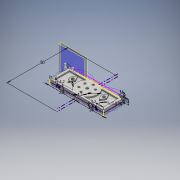
# Autodesk Inventor part: m_mount_l
Saved by Autodesk Inventor 2016 (Build 200138000, 138)
## iProperties
Created: 2016-12-01
Part Number: m_mount_l
Material: 一般
Document SubType Name: Modeling
Designer: KOTA-NPC2
Density: 1 g/cm^3
Appearance: 既定
Author: KOTA-NPC2
Autodesk Inventor part; units mm, degrees
ref_plane "YZ Plane" through (0, 0, 0) normal (1, 0, 0) x (0, 1, 0)
ref_plane "XZ Plane" through (0, 0, 0) normal (0, 1, 0) x (-1, 0, 0)
ref_plane "XY Plane" through (0, 0, 0) normal (0, 0, 1) x (1, 0, 0)
sketch "構築線" plane through (0, 0, 0) normal (0, 0, 1) x (1, 0, 0)
  circle A0 centre (0, 0) radius 8.5
  circle A1 centre (0, 0) radius 2.8 construction
  circle A2 centre (0, 0) radius 5 construction
  line L0 (0, -8.6) -> (-25, -8.6) construction
  line L1 (0, -11.6) -> (-25, -11.6) construction
  circle A3 centre (-12.8148, 0.95) radius 10.05 construction
  circle A4 centre (-12.8148, 0.95) radius 12.55 construction
  circle A5 centre (0, 5) radius 0.8
  circle A6 centre (-4.3301, 2.5) radius 0.8
  circle A7 centre (-4.3301, -2.5) radius 0.8
  circle A8 centre (0, -5) radius 0.8
  circle A9 centre (4.3301, -2.5) radius 0.8
  circle A10 centre (4.3301, 2.5) radius 0.8
  line L2 (25, -8.6) -> (0, -8.6) construction
  circle A11 centre (12.8148, 0.95) radius 10.05 construction
  circle A12 centre (12.8148, 0.95) radius 12.55 construction
  line L3 (0, -11.6) -> (25, -11.6) construction
  line L4 (-22, -8.6) -> (0, -8.6)
  line L5 (0, 25) -> (0, -25)
  line L6 (0, -8.6) -> (22, -8.6)
  circle A13 centre (0, 0) radius 3
  circle A14 centre (0, 0) radius 1
  circle A15 centre (12.8148, 0.95) radius 1.05
  circle A16 centre (-12.8148, 0.95) radius 1.05
  circle A17 centre (12.8148, 0.95) radius 2.75
  circle A18 centre (-12.8148, 0.95) radius 2.75
  line L7 (-4.8008, 7.0144) -> (-17, 7.0144)
  line L8 (4.8008, 7.0144) -> (17, 7.0144)
  line L9 (-4.8008, 7.0144) -> (4.8008, 7.0144)
  line L10 (-17, 7.0144) -> (-22, 7.0144)
  line L11 (-22, 7.0144) -> (-22, -8.6)
  line L12 (22, -8.6) -> (22, 7.0144)
  line L13 (22, 7.0144) -> (17, 7.0144)
  dimension "d22" = 20.1
  dimension "d41" = 20.1
  dimension "d0" = 17
  dimension "d1" = 5.6
  dimension "d2" = 10
  dimension "d12" = 25
  dimension "d13" = 8.6
  dimension "d14" = 0
  dimension "d17" = 0
  dimension "d18" = 25
  dimension "d19" = 3
  dimension "d23" = 25.1
  dimension "d29" = 1.6
  dimension "d30" = 0
  dimension "d31" = 5
  dimension "d34" = 360
  dimension "d38" = 25
  dimension "d42" = 25.1
  dimension "d43" = 25
  dimension "d46" = 22
  dimension "d49" = 50
  dimension "d50" = 25
  dimension "d51" = 25
  dimension "d52" = 22
  dimension "d58" = 6
  dimension "d59" = 2
  dimension "d99" = 2.1
  dimension "d100" = 2.1
  dimension "d105" = 5.5
  dimension "d106" = 5.5
  constraints: 28 end point, 17 centre point, 8 coincident, 8 horizontal, 2 perpendicular, 2 point on circle, 2 tangent, 2 vertical, 1 collinear, 1 concentric, 1 point on line, 23 other
  measures "d0" diameter of A0
  measures "d1" diameter of A1
  measures "d2" diameter of A2
  measures "d12" distance of L0.start L0.end
  measures "d13" distance from line of point (0, 0) L0
  measures "d14" horizontal distance of point (0, 0) L0.start
  measures "d17" horizontal distance of L1.start point (0, 0)
  measures "d18" distance of L1.start L1.end
  measures "d19" distance between parallel lines of L1 L0
  measures "d23" diameter of A4
  measures "d29" diameter of A5
  measures "d30" horizontal distance of point (0, 0) A5.centre
  measures "d31" distance of point (0, 0) A5.centre
  measures "d38" distance of L0.start L2.start
  measures "d42" diameter of A12
  measures "d43" distance of L1.start L3.end
  measures "d46" distance of L0.start L4.start
  measures "d49" distance of L5.start L5.end
  measures "d50" distance of point (0, 0) L5.start
  measures "d51" distance of L5.end point (0, 0)
  measures "d52" distance of L0.start L6.end
  measures "d58" diameter of A13
  measures "d59" diameter of A14
  measures "d99" diameter of A15
  measures "d100" diameter of A16
  measures "d105" diameter of A17
  measures "d106" diameter of A18
extrude "押し出し11" add sketch "構築線" along normal mid plane 4 contours A0 L5 A8 A13 A5 L9 | A0 L8 L13 L12 L6 L5 | L5 L4 L11 L10 L7 A0 | A0 L9 L5 A5 A13 A8 | A13 L5 A14 | L5 A14 A13 | A17 | A18
sketch "模様" plane through (0, 0, 2) normal (0, 0, 1) x (1, 0, 0)
  line L0 (-20, 5.5144) -> (-20, -7.1)
  line L1 (-20, -7.1) -> (20, -7.1) construction
  line L2 (-22, -8.6) -> (-22, 12.4) construction
  line L3 (-22, -8.6) -> (22, -8.6) construction
  line L4 (-20, 5.5144) -> (20, 5.5144) construction
  line L5 (20, 5.5144) -> (20, -7.1)
  line L6 (22, -8.6) -> (22, 12.4) construction
  line L7 (17, 7.0144) -> (-17, 7.0144) construction
  line L8 (-6.4685, 5.5144) -> (-20, 5.5144)
  line L9 (6.4685, 5.5144) -> (20, 5.5144)
  circle A0 centre (-12.8148, 0.95) radius 4 construction
  circle A1 centre (-12.8148, 0.95) radius 1.05 projected
  line L10 (-12.8148, 0.95) -> (-12.8148, 4.95) construction
  line L11 (-12.8148, 0.95) -> (-16.8148, 0.95) construction
  line L12 (-12.8148, 4.95) -> (-15.1242, 0.95)
  line L13 (-15.1242, 0.95) -> (-12.8148, -3.05)
  line L14 (-12.8148, 4.95) -> (-10.5054, 0.95)
  line L15 (-10.5054, 0.95) -> (-12.8148, -3.05)
  circle A2 centre (0, 0) radius 1 projected
  line L16 (-4.6733, -7.1) -> (-20, -7.1)
  line L17 (20, -7.1) -> (4.6733, -7.1)
  circle A3 centre (12.8148, 0.95) radius 4 construction
  circle A4 centre (0, 0) radius 8.5 construction
  arc A5 (-6.4685, 5.5144) -> (-4.6733, -7.1) centre (0, 0) ccw
  circle A6 centre (0, 0) radius 1 projected
  circle A7 centre (12.8148, 0.95) radius 1.05 projected
  arc A8 (4.6733, -7.1) -> (6.4685, 5.5144) centre (0, 0) ccw
  line L18 (12.8148, 0.95) -> (12.8148, 4.95) construction
  line L19 (12.8148, 0.95) -> (8.8148, 0.95) construction
  line L20 (12.8148, 4.95) -> (10.5054, 0.95)
  line L21 (10.5054, 0.95) -> (12.8148, -3.05)
  line L22 (12.8148, -3.05) -> (15.1242, 0.95)
  line L23 (15.1242, 0.95) -> (12.8148, 4.95)
  dimension "d166" = 17
  dimension "d135" = 2
  dimension "d136" = 1.5
  dimension "d137" = 2
  dimension "d138" = 1.5
  dimension "d139" = 8
  dimension "d140" = 60
  dimension "d141" = 60
  dimension "d142" = 60
  dimension "d143" = 60
  dimension "d145" = 8
  dimension "d167" = 60
  dimension "d168" = 60
  dimension "d169" = 60
  constraints: 40 end point, 10 point on circle, 5 point on line, 4 centre point, 4 horizontal, 3 perpendicular, 2 collinear, 2 concentric, 2 vertical, 1 coincident, 1 parallel, 7 other
  measures "d135" distance between parallel lines of L2 L0
  measures "d136" distance between parallel lines of L3 L1
  measures "d137" distance between parallel lines of L6 L5
  measures "d138" distance between parallel lines of L7 L4
  measures "d139" diameter of A0
  measures "d140" angle of L12 L11
  measures "d141" angle of L13 L11
  measures "d142" angle of L14 L12
  measures "d143" angle of L15 L13
  measures "d145" diameter of A3
  measures "d167" angle of L19 L20
  measures "d168" angle of L21 L19
  measures "d169" angle of L22 L21
sketch "スケッチ8" plane through (-22, 7.0144, 2) normal (0, 1, 0) x (1, 0, 0)
  line L0 (44, 0) -> (0, 0) projected
  line L1 (40.5, 0.5) -> (43.5, 0.5)
  line L2 (43.5, 0.5) -> (43.5, 3.5)
  line L3 (43.5, 3.5) -> (40.5, 3.5)
  line L4 (40.5, 3.5) -> (40.5, 0.5)
  line L5 (40.5, 0.5) -> (43.5, 3.5) construction
  line L6 (43.5, 0.5) -> (40.5, 3.5) construction
  point P0 (22, 2)
  point P1 (2, 2)
  point P2 (42, 2)
  dimension "d150" = 3
  dimension "d151" = 3
  dimension "d152" = 0.5
  dimension "d153" = 0.5
  constraints: 12 end point, 2 midpoint, 2 parallel, 1 horizontal, 1 perpendicular
  measures "d150" distance of L3.end L2.end
  measures "d151" distance of L2.end L1.end
  measures "d152" distance from line of L0.start L1
  measures "d153" distance from line of L0.start L2
ref_plane "作業平面2" through (-22, 9.0144, 2) normal (0, 1, 0) x (1, 0, 0)
sketch "スケッチ9" plane through (-22, 9.0144, 2) normal (0, 1, 0) x (1, 0, 0)
  line L0 (44, 0) -> (0, 0) projected
  line L1 (40, 4) -> (44, 4)
  line L2 (44, 4) -> (44, 0)
  line L3 (44, 0) -> (40, 0)
  line L4 (40, 0) -> (40, 4)
  line L5 (40, 4) -> (44, 0) construction
  line L6 (44, 4) -> (40, 0) construction
  point P0 (22, 2)
  point P1 (2, 2)
  point P2 (42, 2)
  dimension "d159" = 2
  dimension "d160" = 4
  dimension "d161" = 4
  dimension "d162" = 2
  dimension "d163" = 2
  constraints: 12 end point, 2 midpoint, 2 parallel, 1 horizontal, 1 perpendicular
  measures "d159" distance from line of L0 point (2, 2)
  measures "d160" distance of L2.end L3.end
  measures "d161" distance of L1.end L2.end
  measures "d162" horizontal distance of L0.start point (42, 2)
  measures "d163" distance from line of L0 point (42, 2)
extrude "押し出し16" cut sketch "模様" against normal blind 1 contours L8 A5 L16 L0 | L5 L17 A8 L9
sketch "固定穴" plane through (0, 0, -2) normal (0, 0, -1) x (-1, 0, 0)
  circle A0 centre (0, 0) radius 8.5
  line L0 (0, -8.6) -> (-25, -8.6) construction
  line L1 (25, -8.6) -> (0, -8.6) construction
  line L2 (0, 25) -> (0, -25)
  circle A1 centre (12.8148, 0.95) radius 2.75
  circle A2 centre (-12.8148, 0.95) radius 2.75
  circle A3 centre (0, 0) radius 1 projected
  circle A4 centre (-12.8148, 0.95) radius 1.05 projected
  circle A5 centre (12.8148, 0.95) radius 1.05 projected
  circle A6 centre (0, 0) radius 2.8
  dimension "d180" = 17
  dimension "d183" = 25
  dimension "d195" = 25
  dimension "d200" = 50
  dimension "d208" = 5.5
  dimension "d209" = 5.5
  dimension "d216" = 5.6
  constraints: 6 end point, 4 centre point, 3 concentric, 2 horizontal, 2 vertical, 1 coincident, 1 collinear
  measures "d180" diameter of A0
  measures "d183" distance of L0.start L0.end
  measures "d195" distance of L0.start L1.start
  measures "d200" distance of L2.start L2.end
  measures "d208" diameter of A1
  measures "d209" diameter of A2
  measures "d216" diameter of A6
extrude "押し出し19" cut sketch "固定穴" against normal blind 2 contours A1 | A2 | A4 | A5
extrude "押し出し20" cut sketch "固定穴" against normal blind 1 contours A0 L2 A6 | L2 A6 A0 | A6 L2 A3 | L2 A3 A6 | A3 L2 | L2 A3
extrude "押し出し21" cut sketch "固定穴" against normal blind 2.1 contours A6 L2 A3 | L2 A3 A6
sketch "ねじ穴+固定(基板)" plane through (-22, -8.6, 2) normal (0, -1, 0) x (1, 0, 0)
  circle A0 centre (38, -2) radius 1
  line L0 (44, -4) -> (44, 0) projected
  line L1 (44, -2) -> (0, -2) construction
  line L2 (0, -4) -> (0, 0) projected
  circle A1 centre (6, -2) radius 1
  line L3 (34.8, -3) -> (32.8, -3)
  line L4 (32.8, -3) -> (32.8, -1)
  line L5 (32.8, -1) -> (34.8, -1)
  line L6 (34.8, -1) -> (34.8, -3)
  line L7 (34.8, -3) -> (32.8, -1) construction
  line L8 (32.8, -3) -> (34.8, -1) construction
  line L9 (11.2, -1) -> (9.2, -1)
  line L10 (9.2, -1) -> (9.2, -3)
  line L11 (9.2, -3) -> (11.2, -3)
  line L12 (11.2, -3) -> (11.2, -1)
  line L13 (11.2, -1) -> (9.2, -3) construction
  line L14 (9.2, -1) -> (11.2, -3) construction
  point P0 (22, -2)
  point P1 (33.8, -2)
  point P2 (33.8, -2)
  point P3 (10.2, -2)
  point P4 (10.2, -2)
  dimension "d219" = 2
  dimension "d220" = 6
  dimension "d221" = 6
  dimension "d222" = 2
  dimension "d223" = 2
  dimension "d224" = 2
  dimension "d225" = 4.2
  dimension "d226" = 2
  dimension "d227" = 2
  dimension "d228" = 4.2
  constraints: 26 end point, 8 midpoint, 4 parallel, 4 point on line, 2 centre point, 2 horizontal, 2 perpendicular
  measures "d219" diameter of A0
  measures "d220" distance from line of L0 A0.centre
  measures "d221" distance from line of L2 A1.centre
  measures "d222" diameter of A1
  measures "d223" distance of L3.start L3.end
  measures "d224" distance of L3.end L4.end
  measures "d225" distance of A0.centre point (33.8, -2)
  measures "d226" distance of L11.end L10.end
  measures "d227" distance of L10.end L9.end
  measures "d228" distance of A1.centre point (10.2, -2)
hole "ねじ穴(基板)" at (16, -8.6, 0) at (-16, -8.6, 0) direction (0, 1, 0) diameter 1.6 depth 3.5 tip angle 118
extrude "押し出し22" add sketch "ねじ穴+固定(基板)" along normal blind 1 contours L3 L4 L5 L6 | L12 L11 L10 L9
fillet "フィレット1" radius 0.5 4 edges at (12.8, -9.1, -1) (12.8, -9.1, 1) (10.8, -9.1, -1) (10.8, -9.1, 1)
fillet "フィレット2" radius 0.5 4 edges at (-12.8, -9.1, -1) (-12.8, -9.1, 1) (-10.8, -9.1, -1) (-10.8, -9.1, 1)
ref_plane "作業平面1" through (-22, 11.0144, 2) normal (0, 1, 0) x (1, 0, 0)
sketch "スケッチ12" plane through (-22, 11.0144, 2) normal (0, 1, 0) x (1, 0, 0)
  circle A0 centre (2, 2) radius 1
  line L0 (0, 0) -> (4, 0) projected
  line L1 (0, 4) -> (0, 0) projected
  circle A1 centre (42, 2) radius 1
  line L2 (44, 0) -> (44, 4) projected
  line L3 (40, 0) -> (44, 0) projected
  point P0 (22, 2)
  dimension "d240" = 2
  dimension "d241" = 2
  dimension "d242" = 2
  dimension "d243" = 2
  dimension "d244" = 2
  dimension "d245" = 2
  constraints: 2 centre point
  measures "d240" diameter of A0
  measures "d241" distance from line of L0 A0.centre
  measures "d242" distance from line of L1 A0.centre
  measures "d243" diameter of A1
  measures "d244" distance from line of L2 A1.centre
  measures "d245" distance from line of L3 A1.centre
hole "穴4" at (20, 11.0144, 0) at (-20, 11.0144, 0) direction (0, -1, 0) diameter 1.6 depth 3.5 tip angle 118
equation "\"d18\" = d12"
